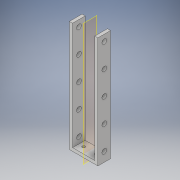
# Autodesk Inventor part: camPostHolderV03
Saved by Autodesk Inventor 2019.4 (Build 234330000, 330)
## iProperties
Created: 2019-04-27
Part Number: camPostHolderV03
Material: Generic
Document SubType Name: Modeling
Designer: steele
Density: 1 g/cm^3
Appearance: Default
Author: steele
Autodesk Inventor part; units mm, degrees
ref_plane "XZ Plane" through (0, 0, 0) normal (0, 1, 0) x (-1, 0, 0)
ref_plane "XY Plane" through (0, 0, 0) normal (0, 0, 1) x (1, 0, 0)
sketch "Sketch1" plane through (0, 0, 0) normal (0, 1, 0) x (-1, 0, 0)
  line L0 (28.575, 12.7) -> (-28.575, 12.7)
  line L1 (-28.575, 12.7) -> (-28.575, -12.7)
  line L2 (-28.575, -12.7) -> (28.575, -12.7)
  line L3 (28.575, -12.7) -> (28.575, 12.7)
  line L4 (28.575, 12.7) -> (-28.575, -12.7) construction
  line L5 (-28.575, 12.7) -> (28.575, -12.7) construction
  point P0 (0, 0)
  dimension "d0" = 57.15
  dimension "d1" = 25.4
  constraints: 12 end point, 2 midpoint, 2 parallel, 1 horizontal, 1 perpendicular
  measures "d0" distance of L0.start L0.end
  measures "d1" distance of L1.end L0.end
extrude "Extrusion1" add sketch "Sketch1" against normal blind 6.35
sketch "Sketch2" plane through (0, 0, 0) normal (0, 1, 0) x (1, 0, 0)
  line L0 (-28.575, -12.7) -> (-28.575, 12.7) projected
  line L1 (-28.575, -12.7) -> (-22.225, -12.7)
  line L2 (-22.225, -12.7) -> (-22.225, 12.7)
  line L3 (-22.225, 12.7) -> (-28.575, 12.7)
  line L4 (-28.575, 12.7) -> (-28.575, -12.7)
  point P0 (0, 0)
  dimension "d4" = 6.35
  constraints: 8 end point, 2 parallel, 1 horizontal, 1 perpendicular
  measures "d4" distance of L3.end L2.end
extrude "Extrusion2" add sketch "Sketch2" along normal blind 215.9
sketch "Sketch5" plane through (-28.575, -6.35, -12.7) normal (-1, 0, 0) x (0, 0, 1)
  circle A0 centre (12.7, 19.05) radius 4.7625
  line L0 (0, 6.35) -> (25.4, 6.35) projected
  line L1 (12.7, 6.35) -> (12.7, 19.05) construction
  circle A1 centre (12.7, 66.675) radius 4.7625
  circle A2 centre (12.7, 114.3) radius 4.7625
  circle A3 centre (12.7, 161.925) radius 4.7625
  circle A4 centre (12.7, 209.55) radius 4.7625
  dimension "d33" = 9.525
  dimension "d34" = 12.7
  dimension "d37" = 47.625
  constraints: 5 centre point, 2 end point, 2 vertical, 8 other
  measures "d33" diameter of A0
  measures "d34" distance from line of L1.end L0
  measures "d37" distance of L1.end A1.centre
extrude "Extrusion5" cut sketch "Sketch5" against normal through all
mirror "Mirror3" about plane through (0, 0, 0) normal (1, 0, 0) of "Extrusion2", "Extrusion5"
sketch "Sketch4" plane through (0, 0, 0) normal (0, 1, 0) x (1, 0, 0)
  point P0 (0, 0)
  point P1 (-12.7, 0)
  point P2 (12.7, 0)
  dimension "d24" = 12.7
  dimension "d25" = 12.7
  measures "d24" distance of point (-12.7, 0) point (0, 0)
  measures "d25" distance of point (12.7, 0) point (0, 0)
hole "Hole1" at (-12.7, 0, 0) at (12.7, 0, 0) direction (0, -1, 0) diameter 5.6134 end through all clearance for "Hex Machine Screw" size "#10" standard "Ansi Unified Screw Threads"
body "Solid1"
